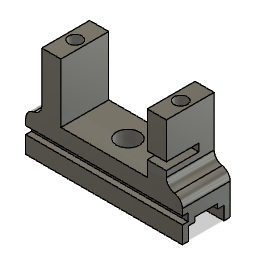
servomount (Autodesk Fusion 360 design; units mm, degrees)
Autodesk Fusion 360 part; units mm, degrees
sketch "Sketch1" plane through (0, 0, 0) normal (0, 1, 0) x (1, 0, 0)
  line L0 (0, 0) -> (41, 0)
  line L1 (41, 0) -> (41, -12.5)
  line L2 (41, -12.5) -> (0, -12.5)
  line L3 (0, -12.5) -> (0, 0)
  dimension "d1" = 41
  dimension "d2" = 12.5
  constraint horizontal L0
  constraint vertical L1
  constraint horizontal L2
  constraint vertical L3
  constraint coincident L0.start L3.end
  measures "d1" distance of L0.start L0.end
  measures "d2" distance of L0.start L2.end
extrude "Extrude1" add sketch "Sketch1" along normal blind 7.2
sketch "Sketch2" plane through (0, 0, 0) normal (0, -1, 0) x (1, 0, 0)
  line L0 (41, 12.5) -> (0, 12.5)
  line L1 (0, 12.5) -> (0, 0)
  line L2 (0, 0) -> (41, 0)
  line L3 (41, 0) -> (41, 12.5)
  line L4 (41, 9.25) -> (0, 9.25)
  line L5 (0, 9.25) -> (0, 3.25)
  line L6 (0, 3.25) -> (41, 3.25)
  line L7 (41, 3.25) -> (41, 9.25)
  dimension "d5" = 6
  constraint horizontal L4
  constraint vertical L5
  constraint horizontal L6
  constraint vertical L7
  constraint coincident L1 L5.end
  constraint coincident L3 L4.start
  constraint midpoint L3 L7
  measures "d5" distance of L4.start L6.end
extrude "Extrude2" cut sketch "Sketch2" against normal blind 1.2 contours L1 L3 L4 L5 L6 L7
sketch "Sketch3" plane through (0, 7.2, 0) normal (0, 1, 0) x (-1, 0, 0)
  line L0 (0, 12.5) -> (-41, 12.5)
  line L1 (-41, 12.5) -> (-41, 0)
  line L2 (-41, 0) -> (0, 0)
  line L3 (0, 0) -> (0, 12.5)
  circle A0 centre (-20.5, 6.25) radius 3
  dimension "d8" = 6
  dimension "d9" = 6.25
  dimension "d10" = 20.5
  measures "d8" diameter of A0
  measures "d9" distance of L2 A0.centre
  measures "d10" distance of L1 A0.centre
extrude "Extrude3" cut sketch "Sketch3" against normal blind 6 contours A0
sketch "Sketch4" plane through (0, 0, 0) normal (0, -1, 0) x (1, 0, 0)
  line L0 (0, 9.25) -> (41, 9.25)
  line L1 (41, 9.25) -> (41, 12.5)
  line L2 (41, 12.5) -> (0, 12.5)
  line L3 (0, 12.5) -> (0, 9.25)
  line L4 (41, 1.625) -> (0, 1.625)
  line L5 (0, 1.625) -> (0, 10.875)
  line L6 (0, 10.875) -> (41, 10.875)
  line L7 (41, 10.875) -> (41, 1.625)
  arc A0 (20.5, 3.25) -> (20.5, 9.25) centre (20.5, 6.25) ccw
  line L8 (20.5, 3.25) -> (41, 3.25)
  line L9 (41, 3.25) -> (41, 9.25)
  line L10 (41, 9.25) -> (20.5, 9.25)
  line L11 (0, 0) -> (41, 0)
  dimension "d13" = 9.25
  dimension "d14" = 1.625
  constraint horizontal L4
  constraint vertical L5
  constraint horizontal L6
  constraint vertical L7
  constraint coincident L3 L5.end
  measures "d13" distance of L4 L6
  measures "d14" distance of L4 L11
sketch "Sketch5" plane through (0, 0, 0) normal (0, -1, 0) x (1, 0, 0)
  line L0 (41, 3.25) -> (0, 3.25)
  line L1 (0, 3.25) -> (0, 0)
  line L2 (0, 0) -> (41, 0)
  line L3 (41, 0) -> (41, 3.25)
sketch "Sketch6" plane through (20.5, 0, 1.625) normal (0, -1, 0) x (1, 0, 0)
  line L0 (20.5, -1.625) -> (-20.5, -1.625)
  line L1 (-20.5, -1.625) -> (-20.5, 0)
  line L2 (-20.5, 0) -> (20.5, 0)
  line L3 (20.5, 0) -> (20.5, -1.625)
  point P0 (20.5, -1.625)
  point P1 (-20.5, 0)
  constraint horizontal L0
  constraint vertical L1
  constraint horizontal L2
  constraint vertical L3
  constraint coincident P1 L1.end
  constraint coincident P0 L0.start
extrude "Extrude4" add sketch "Sketch6" sketch "Sketch4" along normal blind 3.5 of sketch 2 contours L1 L2 L3 L6
sketch "Sketch7" plane through (0, 7.2, 0) normal (0, 1, 0) x (-1, 0, 0)
  circle A0 centre (-20.5, 6.25) radius 3
  line L0 (0, 12.5) -> (-41, 12.5)
  line L1 (-41, 12.5) -> (-41, 0)
  line L2 (-41, 0) -> (0, 0)
  line L3 (0, 0) -> (0, 12.5)
  line L4 (-4.2, 0) -> (-9.2, 0)
  line L5 (-9.2, 0) -> (-9.2, 12.5)
  line L6 (-9.2, 12.5) -> (-4.2, 12.5)
  line L7 (-4.2, 12.5) -> (-4.2, 0)
  line L8 (-36.8, 0) -> (-31.8, 0)
  line L9 (-31.8, 0) -> (-31.8, 12.5)
  line L10 (-31.8, 12.5) -> (-36.8, 12.5)
  line L11 (-36.8, 12.5) -> (-36.8, 0)
  dimension "d17" = 5
  dimension "d18" = 5
  dimension "d19" = 22.6
  dimension "d20" = 4.2
  constraint horizontal L4
  constraint vertical L5
  constraint horizontal L6
  constraint vertical L7
  constraint coincident L0 L5.end
  constraint coincident L2 L4.start
  constraint horizontal L8
  constraint vertical L9
  constraint horizontal L10
  constraint vertical L11
  constraint coincident L2 L8.start
  measures "d17" distance of L4.start L4.end
  measures "d18" distance of L8.start L8.end
  measures "d19" distance of L5 L9
  measures "d20" distance of L1 L11
extrude "Extrude5" add sketch "Sketch7" along normal blind 15.5 contours L0 L2 L4 L5 L6 L7 | L0 L2 L8 L9 L10 L11
sketch "Sketch8" plane through (36.8, 0, 0) normal (1, 0, 0) x (0, 0, -1)
  line L0 (-12.5, 7.2) -> (0, 7.2)
  line L1 (0, 7.2) -> (0, 22.7)
  line L2 (0, 22.7) -> (-12.5, 22.7)
  line L3 (-12.5, 22.7) -> (-12.5, 7.2)
  line L4 (-12.5, 11.2) -> (-4, 11.2)
  line L5 (-4, 11.2) -> (-4, 13.2)
  line L6 (-4, 13.2) -> (-12.5, 13.2)
  line L7 (-12.5, 13.2) -> (-12.5, 11.2)
  dimension "d23" = 8.5
  dimension "d24" = 2
  dimension "d25" = 4
  constraint horizontal L4
  constraint vertical L5
  constraint horizontal L6
  constraint vertical L7
  constraint coincident L3 L4.start
  measures "d23" distance of L4.start L4.end
  measures "d24" distance of L4.start L6.end
  measures "d25" distance of L0 L4
extrude "Extrude6" cut sketch "Sketch8" against normal blind 5 contours L3 L4 L5 L6 L7
fillet "Fillet1" radius 2.5 4 edges at (41, 7.2, 6.25) (36.8, 7.2, 6.25) (0, 7.2, 6.25) (4.2, 7.2, 6.25)
sketch "Sketch9" plane through (0, 22.7, 0) normal (0, 1, 0) x (-1, 0, 0)
  line L0 (-4.2, 12.5) -> (-9.2, 12.5)
  line L1 (-9.2, 12.5) -> (-9.2, 0)
  line L2 (-9.2, 0) -> (-4.2, 0)
  line L3 (-4.2, 0) -> (-4.2, 12.5)
  circle A0 centre (-6.7, 6.25) radius 1.75
  circle A1 centre (-34.3, 6.25) radius 1.75
  line L4 (-31.8, 0) -> (-31.8, 12.5)
  line L5 (-36.8, 0) -> (-31.8, 0)
  dimension "d30" = 3.5
  dimension "d31" = 3.5
  dimension "d32" = 2.5
  dimension "d33" = 2.5
  dimension "d34" = 6.25
  dimension "d35" = 6.25
  measures "d30" diameter of A0
  measures "d31" diameter of A1
  measures "d32" distance of A1.centre L4
  measures "d33" distance of L1 A0.centre
  measures "d34" distance of A1.centre L5
  measures "d35" distance of L2 A0.centre
extrude "Extrude7" cut sketch "Sketch9" against normal blind 4.1 contours A0 | A1
sketch "Sketch10" plane through (0, 0, 12.5) normal (0, 0, 1) x (1, 0, 0)
  arc A0 (2.1, 7.1678) -> (0, 4.7) centre (2.5, 4.7) ccw
  line L0 (0, 4.7) -> (0, -3.5)
  line L1 (0, -3.5) -> (41, -3.5)
  line L2 (41, -3.5) -> (41, 4.7)
  arc A1 (41, 4.7) -> (38.9, 7.1678) centre (38.5, 4.7) ccw
  arc A2 (36.8, 9.6356) -> (38.9, 7.1678) centre (39.3, 9.6356) ccw
  line L3 (36.8, 9.6356) -> (36.8, 11.2)
  line L4 (36.8, 11.2) -> (31.8, 11.2)
  line L5 (31.8, 11.2) -> (31.8, 7.2)
  line L6 (31.8, 7.2) -> (9.2, 7.2)
  line L7 (9.2, 7.2) -> (9.2, 22.7)
  line L8 (9.2, 22.7) -> (4.2, 22.7)
  line L9 (4.2, 22.7) -> (4.2, 9.6356)
  arc A3 (2.1, 7.1678) -> (4.2, 9.6356) centre (1.7, 9.6356) ccw
  line L10 (41, 1) -> (0, 1)
  line L11 (0, 1) -> (0, 3)
  line L12 (0, 3) -> (41, 3)
  line L13 (41, 3) -> (41, 1)
  dimension "d38" = 2
  dimension "d39" = 4.5
  constraint horizontal L10
  constraint vertical L11
  constraint horizontal L12
  constraint vertical L13
  constraint coincident L0 L11.end
  constraint coincident L2 L10.start
  measures "d38" distance of L10 L12
  measures "d39" distance of L1 L10
extrude "Extrude8" cut sketch "Sketch10" against normal blind 1.5 contours L0 L2 L10 L11 L12 L13
equation "d3 = 6 mm + 1.2 mm"
equation "d9 = ( 12.5 / 2 ) * 1 mm"
equation "d10 = ( 41 / 2 ) * 1 mm"
equation "d14 = ( 12.5 mm - d13 ) / 2"
equation "d20 = ( ( 41 - 32.6 ) / 2 ) * 1 mm"
equation "d25 = 5 mm - d24 / 2"
equation "d34 = ( 12.5 / 2 ) * 1 mm"
equation "d35 = d34"
equation "d39 = 2.5 mm + 2 mm"
named bodies: "servomount"
